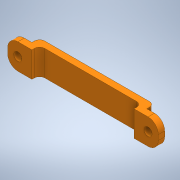
# Autodesk Inventor part: battery_mount_1s_500mah
Saved by Autodesk Inventor 2020 (Build 240168000, 168)
## iProperties
Created: 2016-10-05
Part Number: battery_mount_1s_500mah
Material: Generic
Document SubType Name: Modeling
Designer: Luke
Density: 1 g/cm^3
Appearance: Orange
Author: Luke
Autodesk Inventor part; units mm, degrees
ref_plane "YZ Plane" through (0, 0, 0) normal (1, 0, 0) x (0, 1, 0)
ref_plane "XZ Plane" through (0, 0, 0) normal (0, 1, 0) x (-1, 0, 0)
sketch "Sketch1" plane through (0, 0, 0) normal (0, 1, 0) x (-1, 0, 0)
  line L0 (0, 0) -> (-45, 0)
  line L1 (-45, 0) -> (-45, -10)
  line L2 (-45, -10) -> (0, -10)
  line L3 (0, -10) -> (0, 0)
  dimension "d0" = 10
  dimension "d1" = 45
  constraints: 8 end point, 2 parallel, 1 horizontal, 1 perpendicular
  measures "d0" distance of L2.end L0.start
  measures "d1" distance of L1.end L2.end
extrude "Extrusion1" add sketch "Sketch1" along normal blind 2.5
sketch "Sketch2" plane through (0, 0, 0) normal (0, -1, 0) x (1, 0, 0)
  line L0 (0, 0) -> (45, 0) projected
  line L1 (0, -10) -> (0, 0) projected
  line L2 (45, -10) -> (0, -10) projected
  line L3 (45, 0) -> (45, -10) projected
  line L4 (0, 0) -> (45, 0) projected
  line L5 (2.5, 0) -> (2.5, -10)
  line L6 (42.5, 0) -> (42.5, -10)
  line L7 (45, -10) -> (0, -10) projected
  dimension "d4" = 2.5
  dimension "d5" = 2.5
  constraints: 4 end point, 4 point on line, 1 perpendicular, 1 vertical
  measures "d4" distance between parallel lines of L5 L1
  measures "d5" distance between parallel lines of L3 L6
extrude "Extrusion2" add sketch "Sketch2" along normal blind 3 contours L0 L5 L2 L1 | L0 L3 L2 L6
sketch "Sketch3" plane through (0, -3, 0) normal (0, -1, 0) x (1, 0, 0)
  line L0 (0, -10) -> (2.5, -10) projected
  line L1 (2.5, -10) -> (2.5, 0) projected
  line L2 (2.5, 0) -> (0, 0) projected
  line L3 (0, 0) -> (0, -10) projected
  line L4 (0, 0) -> (-7, 0)
  line L5 (-7, 0) -> (-7, -10)
  line L6 (-7, -10) -> (0, -10)
  line L7 (0, -10) -> (0, 0)
  line L8 (0, -10) -> (2.5, -10) projected
  dimension "d8" = 7
  constraints: 8 end point, 2 parallel, 2 perpendicular, 1 horizontal
  measures "d8" distance of L2.end L4.end
extrude "Extrusion3" add sketch "Sketch3" against normal blind 2.5 contours L6 L5 L4 L3
sketch "Sketch4" plane through (0, -0.5, 0) normal (0, 1, 0) x (1, 0, 0)
  line L0 (-7, 0) -> (0, 0) projected
  line L1 (0, 10) -> (0, 0) projected
  line L2 (0, 10) -> (-7, 10) projected
  line L3 (-7, 10) -> (-7, 0) projected
  line L4 (0, 10) -> (0, 0) construction
  line L5 (0, 5) -> (-3, 5) construction
  circle A0 centre (-3, 5) radius 1.6
  dimension "d11" = 3
  dimension "d12" = 3.2
  constraints: 2 end point, 1 centre point, 1 coincident, 1 horizontal, 1 midpoint
  measures "d11" distance of L5.start L5.end
  measures "d12" diameter of A0
extrude "Extrusion4" cut sketch "Sketch4" against normal up to surface (2.5 mm away) contours A0
ref_plane "Work Plane1" through (22.5, 0, 0) normal (1, 0, 0) x (0, 0, -1)
fillet "Fillet1" radius 4 2 edges at (-7, -1.75, 0) (-7, -1.75, -10)
mirror "Mirror1" about plane through (22.5, 0, 0) normal (1, 0, 0) of "Fillet1", "Extrusion4", "Extrusion3"
fillet "Fillet3" radius 2 4 edges at (2.5, 0, -5) (42.5, 0, -5) (0, 2.5, -5) (45, 2.5, -5)
equation "\"d2\" = wall_thickness"
equation "\"d4\" = wall_thickness"
equation "\"d5\" = wall_thickness"
equation "\"d9\" = wall_thickness"
equation "\"d13\" = wall_thickness"
equation "\"wall_thickness\" = 2.5"
body "Solid1"
